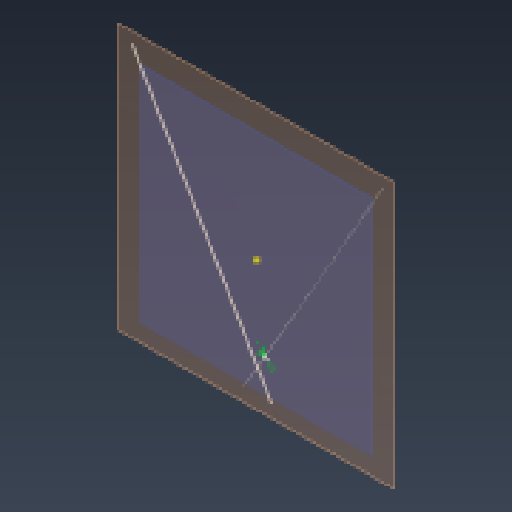
# Autodesk Inventor part: Задняя панель
Saved by Autodesk Inventor 2023.2 (Build 272271030, 271C)
## iProperties
Created: 2025-08-26
Part Number: Задняя панель
Material: Типовые
Document SubType Name: Modeling
Designer: Олег Коноваленко
Density: 1 g/cm^3
Appearance: Синий — малярная краска — глянцевая
Author: Олег Коноваленко
Autodesk Inventor part; units mm, degrees
ref_plane "YZ Plane" through (0, 0, 0) normal (1, 0, 0) x (0, 1, 0)
ref_plane "XZ Plane" through (0, 0, 0) normal (0, 1, 0) x (-1, 0, 0)
sketch "Эскиз1" plane through (0, 0, 0) normal (0, 0, 1) x (1, 0, 0)
  line L0 (200, -193) -> (-200, -193)
  line L1 (-200, -193) -> (-200, 193)
  line L2 (-200, 193) -> (200, 193)
  line L3 (200, 193) -> (200, -193)
  line L4 (200, -193) -> (-200, 193) construction
  line L5 (-200, -193) -> (200, 193) construction
  point P0 (0, 0)
  dimension "d0" = 400
  dimension "d1" = 386
  constraints: 12 end point, 2 midpoint, 2 parallel, 1 horizontal, 1 perpendicular
  measures "d0" distance of L0.start L0.end
  measures "d1" distance of L0.end L1.end
extrude "Выдавливание1" add sketch "Эскиз1" along normal mid plane 4
sketch "Эскиз2" plane through (0, 0, -2) normal (0, 0, -1) x (-1, 0, 0)
  line L0 (-217.6269, 215.5345) -> (23.8731, -202.7558) construction
  line L1 (-23.8731, -202.7558) -> (217.6269, 215.5345) construction
  line L2 (-7.186, -135.2399) -> (-19.0679, -142.0999) construction
  circle A0 centre (-13.1269, -138.6699) radius 2
  line L3 (-24.686, -104.929) -> (-36.5679, -111.789) construction
  circle A1 centre (-30.6269, -108.359) radius 2
  line L4 (-42.186, -74.6181) -> (-54.0679, -81.4781) construction
  circle A2 centre (-48.1269, -78.0481) radius 2
  line L5 (-59.686, -44.3072) -> (-71.5679, -51.1672) construction
  circle A3 centre (-65.6269, -47.7372) radius 2
  line L6 (-77.186, -13.9963) -> (-89.0679, -20.8563) construction
  circle A4 centre (-83.1269, -17.4263) radius 2
  line L7 (-94.686, 16.3146) -> (-106.5679, 9.4546) construction
  circle A5 centre (-100.6269, 12.8846) radius 2
  line L8 (-112.186, 46.6255) -> (-124.0679, 39.7655) construction
  circle A6 centre (-118.1269, 43.1955) radius 2
  line L9 (-129.686, 76.9364) -> (-141.5679, 70.0764) construction
  circle A7 centre (-135.6269, 73.5064) radius 2
  line L10 (-147.186, 107.2472) -> (-159.0679, 100.3872) construction
  circle A8 centre (-153.1269, 103.8172) radius 2
  line L11 (-164.686, 137.5581) -> (-176.5679, 130.6981) construction
  circle A9 centre (-170.6269, 134.1281) radius 2
  line L12 (7.186, -135.2399) -> (19.0679, -142.0999) construction
  circle A10 centre (13.1269, -138.6699) radius 2
  circle A11 centre (30.6269, -108.359) radius 2
  circle A12 centre (48.1269, -78.0481) radius 2
  circle A13 centre (65.6269, -47.7372) radius 2
  circle A14 centre (83.1269, -17.4263) radius 2
  circle A15 centre (100.6269, 12.8846) radius 2
  circle A16 centre (118.1269, 43.1955) radius 2
  circle A17 centre (135.6269, 73.5064) radius 2
  circle A18 centre (153.1269, 103.8172) radius 2
  circle A19 centre (170.6269, 134.1281) radius 2
  point P0 (0, 0)
  dimension "d4" = 4
  dimension "d7" = 35
  dimension "d12" = 4
  dimension "d15" = 35
  constraints: 26 end point, 20 centre point, 2 midpoint, 2 point on line, 77 other
  measures "d4" diameter of A0
  measures "d7" distance of L2.start L3.start
  measures "d12" diameter of A10
  measures "d15" distance of A10.centre A11.centre
extrude "Выдавливание2" cut sketch "Эскиз2" against normal up to next
